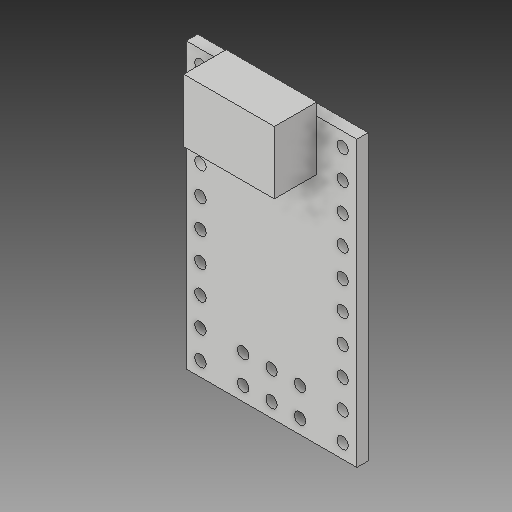
# Autodesk Inventor part: Pololu_A_Star_32U4_Micro
Saved by Autodesk Inventor 2018.1 (Build 221171000, 171)
## iProperties
Part Number: Pololu_A_Star_32U4_Micro
Material: 一般
Document SubType Name: Modeling
Designer: sktom
Density: 1 g/cm^3
Appearance: 既定
Author: sktom
Autodesk Inventor part; units mm, degrees
ref_plane "YZ Plane" through (0, 0, 0) normal (1, 0, 0) x (0, 1, 0)
ref_plane "XZ Plane" through (0, 0, 0) normal (0, 1, 0) x (-1, 0, 0)
ref_plane "XY Plane" through (0, 0, 0) normal (0, 0, 1) x (1, 0, 0)
sketch "スケッチ1" plane through (0, 0, 0) normal (0, 0, 1) x (1, 0, 0)
  line L0 (-7.62, -12.7) -> (7.62, -12.7)
  line L1 (7.62, -12.7) -> (7.62, 12.7)
  line L2 (7.62, 12.7) -> (-7.62, 12.7)
  line L3 (-7.62, 12.7) -> (-7.62, -12.7)
  line L4 (-7.62, -12.7) -> (7.62, 12.7) construction
  line L5 (7.62, -12.7) -> (-7.62, 12.7) construction
  point P0 (0, 0)
  dimension "d0" = 15.24
  dimension "d1" = 25.4
  constraints: 12 end point, 2 midpoint, 2 parallel, 1 horizontal, 1 perpendicular
  measures "d0" distance of L2.end L1.end
  measures "d1" distance of L0.end L1.end
extrude "押し出し1" add sketch "スケッチ1" along normal blind 1.02
sketch "スケッチ2" plane through (0, 0, 1.02) normal (0, 0, 1) x (1, 0, 0)
  line L0 (-6.35, -11.43) -> (6.35, -11.43) construction
  line L1 (6.35, -11.43) -> (6.35, 11.43) construction
  line L2 (6.35, 11.43) -> (-6.35, 11.43) construction
  line L3 (-6.35, 11.43) -> (-6.35, -11.43) construction
  line L4 (-6.35, -11.43) -> (6.35, 11.43) construction
  line L5 (6.35, -11.43) -> (-6.35, 11.43) construction
  line L6 (7.62, 12.7) -> (-7.62, 12.7) construction
  circle A0 centre (-6.35, 11.43) radius 0.51
  circle A1 centre (-6.35, 8.89) radius 0.51
  circle A2 centre (-6.35, 6.35) radius 0.51
  circle A3 centre (-6.35, 3.81) radius 0.51
  circle A4 centre (-6.35, 1.27) radius 0.51
  circle A5 centre (-6.35, -1.27) radius 0.51
  circle A6 centre (-6.35, -3.81) radius 0.51
  circle A7 centre (-6.35, -6.35) radius 0.51
  circle A8 centre (-6.35, -8.89) radius 0.51
  circle A9 centre (-6.35, -11.43) radius 0.51
  circle A10 centre (6.35, 11.43) radius 0.51
  circle A11 centre (6.35, 8.89) radius 0.51
  circle A12 centre (6.35, 6.35) radius 0.51
  circle A13 centre (6.35, 3.81) radius 0.51
  circle A14 centre (6.35, 1.27) radius 0.51
  circle A15 centre (6.35, -1.27) radius 0.51
  circle A16 centre (6.35, -3.81) radius 0.51
  circle A17 centre (6.35, -6.35) radius 0.51
  circle A18 centre (6.35, -8.89) radius 0.51
  circle A19 centre (6.35, -11.43) radius 0.51
  line L7 (-2.54, -11.43) -> (2.54, -11.43) construction
  line L8 (2.54, -11.43) -> (2.54, -8.89) construction
  line L9 (2.54, -8.89) -> (-2.54, -8.89) construction
  line L10 (-2.54, -8.89) -> (-2.54, -11.43) construction
  circle A20 centre (-2.54, -8.89) radius 0.51
  circle A21 centre (-2.54, -11.43) radius 0.51
  circle A22 centre (0, -8.89) radius 0.51
  circle A23 centre (0, -11.43) radius 0.51
  circle A24 centre (2.54, -8.89) radius 0.51
  circle A25 centre (2.54, -11.43) radius 0.51
  point P0 (0, 0)
  dimension "d4" = 12.7
  dimension "d5" = 1.27
  dimension "d6" = 1.02
  dimension "d9" = 2.54
  dimension "d12" = 12.7
  dimension "d15" = 3.81
  dimension "d16" = 5.08
  dimension "d19" = 2.54
  dimension "d22" = 2.54
  constraints: 26 centre point, 20 end point, 4 horizontal, 4 parallel, 2 midpoint, 2 perpendicular, 2 vertical, 1 coincident, 1 equal radius, 1 horizontal alignment, 1 point on line, 48 other
  measures "d4" distance of L1.end L2.end
  measures "d5" distance between parallel lines of L6 L2
  measures "d6" diameter of A0
  measures "d9" distance of L2.end A1.centre
  measures "d12" distance of L2.end A10.centre
  measures "d15" distance from line of A8.centre L10
  measures "d16" distance of L8.end L9.end
  measures "d19" distance of A20.centre A21.centre
  measures "d22" distance of A20.centre A22.centre
extrude "押し出し2" cut sketch "スケッチ2" against normal blind 1.02
sketch "スケッチ3" plane through (0, 0, 1.02) normal (0, 0, 1) x (1, 0, 0)
  line L0 (-4.05, 8.2) -> (4.05, 8.2)
  line L1 (4.05, 8.2) -> (4.05, 13.8)
  line L2 (4.05, 13.8) -> (-4.05, 13.8)
  line L3 (-4.05, 13.8) -> (-4.05, 8.2)
  line L4 (-7.62, -12.7) -> (7.62, -12.7) projected
  point P0 (0, 0)
  point P1 (0, 8.2)
  dimension "d27" = 26.5
  dimension "d28" = 8.1
  dimension "d29" = 5.6
  constraints: 8 end point, 2 parallel, 1 horizontal, 1 midpoint, 1 perpendicular, 1 vertical alignment
  measures "d27" distance between parallel lines of L2 L4
  measures "d28" distance of L1.end L2.end
  measures "d29" distance of L0.end L1.end
extrude "押し出し3" add sketch "スケッチ3" along normal blind 3.8
